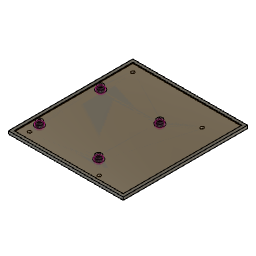
baseplate (Autodesk Fusion 360 design; units mm, degrees)
Autodesk Fusion 360 part; units mm, degrees
sketch "Sketch1" plane through (0, 0, 0) normal (0, 0, 1) x (1, 0, 0) in component "PCB"
  line L0 (35.5, 37) -> (-35.5, 37)
  line L1 (-35.5, 37) -> (-35.5, -37)
  line L2 (-35.5, -37) -> (35.5, -37)
  line L3 (35.5, -37) -> (35.5, 37)
  line L4 (35.5, 37) -> (-35.5, -37) construction
  line L5 (-35.5, 37) -> (35.5, -37) construction
  line L6 (31, 32) -> (-31, 32) construction
  line L7 (-31, 32) -> (-31, -32) construction
  line L8 (-31, -32) -> (31, -32) construction
  line L9 (31, -32) -> (31, 32) construction
  line L10 (31, 32) -> (-31, -32) construction
  line L11 (-31, 32) -> (31, -32) construction
  circle A0 centre (-31, 32) radius 1.5
  circle A1 centre (31, 32) radius 1.5
  circle A2 centre (31, -32) radius 1.5
  circle A3 centre (-31, -32) radius 1.5
  dimension "d1" = 71
  dimension "d2" = 74
  dimension "d3" = 62
  dimension "d4" = 64
  dimension "d5" = 3
  dimension "d6" = 3
  dimension "d7" = 3
  dimension "d8" = 3
  constraint perpendicular L0 L1
  constraint parallel L0 L2
  constraint parallel L1 L3
  constraint horizontal L0
  constraint coincident L4 origin
  constraint coincident L5 origin
  constraint perpendicular L6 L7
  constraint parallel L6 L8
  constraint parallel L7 L9
  constraint horizontal L6
  constraint coincident L10 origin
  constraint coincident L11 origin
  constraint coincident L6.end L7.start
  constraint coincident L6.start L9.end
  constraint coincident L8.end L9.start
  constraint coincident L7.end L8.start
  measures "d1" distance of L1.end L2.end
  measures "d2" distance of L0.end L1.end
  measures "d3" distance of L7.end L8.end
  measures "d4" distance of L6.end L7.end
  measures "d5" diameter of A0
  measures "d6" diameter of A1
  measures "d7" diameter of A2
  measures "d8" diameter of A3
form "Form1" [no effect] in component "7 segment display"
extrude "Extrude1" add sketch "Sketch1" along normal blind 1.57 sketch seen with x (1, 0, 0) y (0, 1, 0) z (0, 0, 1) at (35.5, 37, 0) makes body 1 in component "Board"
mesh "Mesh1" [no effect] in component "7 segment display"
mesh "Mesh1'" [no effect] in component "PSU"
mesh "Mesh1''" [no effect] in component "PCB"
mesh "Mesh2" [no effect] in component "PCB"
mesh "Mesh3" [no effect] in component "PCB"
mesh "Mesh4" [no effect] in component "PCB"
sketch "Plate" plane through (0, 0, 0) normal (0, 0, 1) x (1, 0, 0) in component "Baseplate"
  line L0 (60, 65) -> (-60, 65)
  line L1 (-60, 65) -> (-60, -65)
  line L2 (-60, -65) -> (60, -65)
  line L3 (60, -65) -> (60, 65)
  line L4 (60, 65) -> (-60, -65) construction
  line L5 (-60, 65) -> (60, -65) construction
  dimension "d19" = 120
  dimension "d20" = 130
  constraint perpendicular L0 L1
  constraint parallel L0 L2
  constraint parallel L1 L3
  constraint horizontal L0
  constraint coincident L4 origin
  constraint coincident L5 origin
  measures "d19" distance of L1.end L2.end
  measures "d20" distance of L0.end L1.end
extrude "Extrude1'" add sketch "Plate" along normal blind 2 separate body makes body 2 in component "Baseplate"
mesh "Mesh1'''" [no effect] in component "IEC320"
sketch "Rand" plane through (0, 0, 2) normal (0, 0, 1) x (-1, 0, 0) in component "Baseplate"
  line L0 (-60, 65) -> (-60, -65)
  line L1 (-60, -65) -> (60, -65)
  line L2 (60, -65) -> (60, 65)
  line L3 (60, 65) -> (-60, 65)
  line L4 (-57, 62) -> (-57, -62)
  line L5 (-57, -62) -> (57, -62)
  line L6 (57, -62) -> (57, 62)
  line L7 (57, 62) -> (-57, 62)
  dimension "d29" = -3
extrude "Extrude3" add sketch "Rand" along normal blind 1 bodies 2 in component "Baseplate"
sketch "Holes" plane through (0, 0, 2) normal (0, 0, 1) x (-1, 0, 0) in component "Baseplate"
  line L0 (-57, 62) -> (-57, -62)
  line L1 (-57, -62) -> (57, -62)
  line L2 (57, -62) -> (57, 62)
  line L3 (57, 62) -> (-57, 62)
  circle A0 centre (-27, 57) radius 1.75
  line L4 (-57, -62) -> (-57, 62)
  circle A1 centre (-37.4984, -40.0244) radius 1.75
  circle A2 centre (49, 54) radius 1.75
  circle A3 centre (49, -54) radius 1.75
  dimension "d32" = 3.5
  dimension "d33" = 5
  dimension "d34" = 30
  dimension "d35" = 3.5
  dimension "d36" = 21.9756
  dimension "d37" = 19.5016
  dimension "d38" = 3.5
  dimension "d39" = 8
  dimension "d40" = 8
  dimension "d41" = 3.5
  dimension "d42" = 8
  dimension "d43" = 8
  measures "d32" diameter of A0
  measures "d33" distance of L3 A0.centre
  measures "d34" distance of A0.centre L4
  measures "d35" diameter of A1
  measures "d36" distance of L1 A1.centre
  measures "d37" distance of L4 A1.centre
  measures "d38" diameter of A2
  measures "d39" distance of L2 A2.centre
  measures "d40" distance of L3 A2.centre
  measures "d41" diameter of A3
  measures "d42" distance of L1 A3.centre
  measures "d43" distance of L2 A3.centre
extrude "Extrude4" cut sketch "Holes" against normal up to surface (2 mm away) contours A0 | A1 | A2 | A3 bodies 2 in component "Baseplate"
sketch "Sketch1 (2)" plane through (0, 0, 0) normal (0, 0, -1) x (1, 0, 0) in component "Standoffs"
  circle A0 centre (27, 57) radius 1.75
  circle A1 centre (-49, 54) radius 1.75
  circle A2 centre (37.4984, -40.0244) radius 1.75
  circle A3 centre (-49, -54) radius 1.75
  line L0 (60, -65) -> (60, 65)
  line L1 (60, 65) -> (-60, 65)
  line L2 (-60, 65) -> (-60, -65)
  line L3 (-60, -65) -> (60, -65)
  circle A4 centre (-49, -54) radius 4
  circle A5 centre (37.4984, -40.0244) radius 4
  circle A6 centre (27, 57) radius 4
  circle A7 centre (-49, 54) radius 4
  dimension "d46" = 8
  dimension "d47" = 8
  dimension "d48" = 8
  dimension "d49" = 8
  constraint concentric A3 A4
  constraint concentric A2 A5
  constraint concentric A0 A6
  constraint concentric A1 A7
  measures "d46" diameter of A4
  measures "d47" diameter of A5
  measures "d48" diameter of A6
  measures "d49" diameter of A7
extrude "Extrude1''" add sketch "Sketch1 (2)" along normal blind 6 separate body contours A4 | A5 | A6 | A7 makes body 3 at (30.995, -56.8006, -4) makes body 4 at (-45.005, 54.1994, -4) makes body 5 at (-45.005, -53.8006, -4) makes body 6 at (41.4934, 40.2238, -4) in component "Standoffs"
sketch "PCB standoffs" plane through (0, 0, 2) normal (0, 0, 1) x (-1, 0, 0) in component "Baseplate"
  circle A0 centre (-27, 57) radius 1.75
  circle A1 centre (49, 54) radius 1.75
  circle A2 centre (-37.4984, -40.0244) radius 1.75
  circle A3 centre (49, -54) radius 1.75
  line L0 (-57, 62) -> (-57, -62)
  line L1 (-57, -62) -> (57, -62)
  line L2 (57, -62) -> (57, 62)
  line L3 (57, 62) -> (-57, 62)
  circle A4 centre (50.109, -21.4767) radius 1.5
  circle A5 centre (-11.891, -21.4767) radius 1.5
  circle A6 centre (-11.891, 42.5233) radius 1.5
  circle A7 centre (50.109, 42.5233) radius 1.5
  circle A8 centre (50.109, 42.5233) radius 3
  circle A9 centre (50.109, -21.4767) radius 3
  circle A10 centre (-11.891, -21.4767) radius 3
  circle A11 centre (-11.891, 42.5233) radius 3
  circle A12 centre (50.109, -21.4767) radius 1.35
  circle A13 centre (-11.891, -21.4767) radius 1.35
  circle A14 centre (50.109, 42.5233) radius 1.35
  circle A15 centre (-11.891, 42.5233) radius 1.35
  dimension "d52" = 6
  dimension "d53" = 6
  dimension "d54" = 6
  dimension "d55" = 6
  dimension "d59" = 2.7
  dimension "d60" = 2.7
  dimension "d61" = 2.7
  dimension "d62" = 2.7
  constraint concentric A7 A8
  constraint concentric A4 A9
  constraint concentric A5 A10
  constraint concentric A6 A11
  constraint concentric A9 A12
  constraint concentric A10 A13
  constraint concentric A8 A14
  constraint concentric A11 A15
  measures "d52" diameter of A8
  measures "d53" diameter of A9
  measures "d54" diameter of A10
  measures "d55" diameter of A11
  measures "d59" diameter of A12
  measures "d60" diameter of A13
  measures "d61" diameter of A14
  measures "d62" diameter of A15
extrude "Extrude6" add sketch "PCB standoffs" along normal blind 4 contours A4 | A5 | A6 | A7 | A8 | A9 | A10 | A11 bodies 2 in component "Baseplate"
chamfer "Chamfer3" distance 1.5 angle 45 4 edges at (14.688, -43.6081, 2) (-47.312, -43.6081, 2) (-47.312, 20.3919, 2) (14.688, 20.3919, 2) on bodies 2 in component "Baseplate"
sketch "Outer" plane through (0, 0, 2) normal (0, 0, 1) x (-1, 0, 0) in component "Feet"
  circle A0 centre (0, 0) radius 10
  dimension "d66" = 20
  constraint coincident A0.centre origin
  measures "d66" diameter of A0
extrude "Extrude1'''" add sketch "Outer" along normal blind 5 separate body makes body 7 in component "Feet"
fillet "Fillet1" radius 1.5 1 edges at (9.3233, 3.6162, 7) on bodies 7 in component "Feet"
sketch "Inner" plane through (0, 0, 7) normal (0, 0, 1) x (-1, 0, 0) in component "Feet"
  circle A0 centre (0, 0) radius 8.5
  circle A1 centre (0, 0) radius 4
  dimension "d70" = 8
  constraint coincident A0.centre A1.centre
  measures "d70" diameter of A1
extrude "Extrude2" cut sketch "Inner" against normal blind 3 contours A1 bodies 7 in component "Feet"
sketch "Hole" plane through (0, 0, 4) normal (0, 0, 1) x (-1, 0, 0) in component "Feet"
  circle A0 centre (0, 0) radius 4
  circle A1 centre (0, 0) radius 1.6
  dimension "d73" = 3.2
  constraint concentric A0 A1
  measures "d73" diameter of A1
extrude "Extrude3'" cut sketch "Hole" against normal up to surface (2 mm away) contours A1 bodies 7 in component "Feet"
component "Baseplate" placed x (1, 0, 0) y (0, 1, 0) z (0, 0, 1) at (0, 0, 0)
component "PCB" placed x (1, 0, 0) y (0, 1, 0) z (0, 0, 1) at (-19.109, -10.5233, 5.7467)
component "7 segment display" placed x (1, 0, 0) y (0, 1, 0) z (0, 0, 1) at (0, 0, 0)
component "PSU" placed x (-1, 0, 0) y (0, -1, 0) z (0, 0, 1) at (-143, 21, 0)
component "IEC320" placed x (1, 0, 0) y (0, 1, 0) z (0, 0, 1) at (0, 0, 0)
component "Standoffs" placed x (1, 0, 0) y (0, 1, 0) z (0, 0, 1) at (0, 0, 0)
component "Feet" placed x (1, 0, 0) y (0, 1, 0) z (0, 0, 1) at (0, 0, 0)
component "Board" placed x (1, 0, 0) y (0, 1, 0) z (0, 0, 1) at (-35.5, -37, 0) in component "PCB"
named bodies: "Board"
